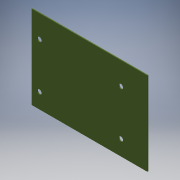
# Autodesk Inventor part: main_pcb
Saved by Autodesk Inventor 2018 (Build 220112000, 112)
## iProperties
Created: 2018-04-09
Part Number: main_pcb
Material: ガラス
Document SubType Name: Modeling
Designer: NaMACHAN
Density: 2.18 g/cm^3
Appearance: オリーブ グリーン
Author: NaMACHAN
Autodesk Inventor part; units mm, degrees
ref_plane "YZ Plane" through (0, 0, 0) normal (1, 0, 0) x (0, 1, 0)
ref_plane "XZ Plane" through (0, 0, 0) normal (0, 1, 0) x (-1, 0, 0)
ref_plane "XY Plane" through (0, 0, 0) normal (0, 0, 1) x (1, 0, 0)
sketch "スケッチ1" plane through (0, 0, 0) normal (0, 1, 0) x (-1, 0, 0)
  line L0 (-38.735, -27.94) -> (38.735, -27.94)
  line L1 (38.735, -27.94) -> (38.735, 27.94)
  line L2 (38.735, 27.94) -> (-38.735, 27.94)
  line L3 (-38.735, 27.94) -> (-38.735, -27.94)
  line L4 (-38.735, -27.94) -> (38.735, 27.94) construction
  line L5 (38.735, -27.94) -> (-38.735, 27.94) construction
  point P0 (0, 0)
  dimension "d0" = 77.47
  dimension "d1" = 55.88
  constraints: 12 end point, 2 midpoint, 2 parallel, 1 horizontal, 1 perpendicular
  measures "d0" distance of L2.end L1.end
  measures "d1" distance of L1.end L0.end
extrude "押し出し1" add sketch "スケッチ1" along normal blind 0.6
sketch "スケッチ2" plane through (0, 0.6, 0) normal (0, 1, 0) x (1, 0, 0)
  line L0 (-38.735, -27.94) -> (38.735, -27.94) projected
  line L1 (-38.735, 27.94) -> (-38.735, -27.94) projected
  point P0 (0, 0)
  point P1 (-34.854, -11.43)
  point P2 (-34.854, 18.57)
  point P3 (35.146, 18.57)
  point P4 (35.146, -11.43)
  dimension "d4" = 16.51
  dimension "d5" = 3.881
  dimension "d15" = 30
  dimension "d16" = 70
  constraints: 2 horizontal alignment, 2 vertical alignment
  measures "d4" distance from line of L0 point (-34.854, -11.43)
  measures "d5" distance from line of L1 point (-34.854, -11.43)
  measures "d15" distance of point (-34.854, 18.57) point (-34.854, -11.43)
  measures "d16" distance of point (35.146, -11.43) point (-34.854, -11.43)
hole "穴1" at (-34.854, 0.6, 11.43) at (-34.854, 0.6, -18.57) at (35.146, 0.6, -18.57) at (35.146, 0.6, 11.43) direction (0, -1, 0) diameter 3 end through all
